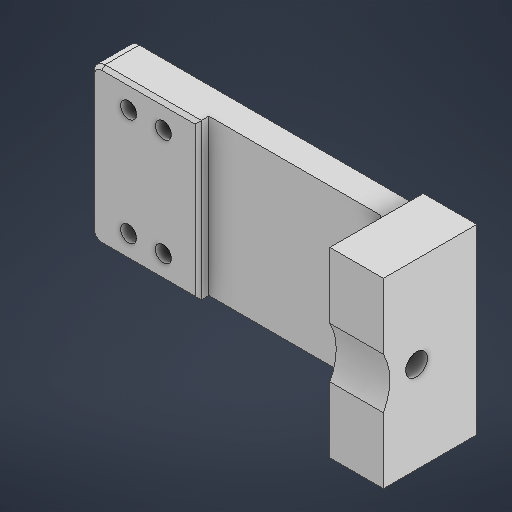
# Autodesk Inventor part: tool4_2
Saved by Autodesk Inventor 2027.1 (Build 311270010, 270A)
## iProperties
Created: 2026-08-16
Part Number: tool4_2
Material: Generic
Document SubType Name: Sheet Metal
Designer: MSI
Density: 1 g/cm^3
Sheet Metal Rule: Default_mm
Appearance: Default
Author: MSI
Autodesk Inventor part; units mm, degrees
ref_plane "YZ Plane" through (0, 0, 0) normal (1, 0, 0) x (0, 1, 0)
ref_plane "XZ Plane" through (0, 0, 0) normal (0, 1, 0) x (-1, 0, 0)
ref_plane "XY Plane" through (0, 0, 0) normal (0, 0, 1) x (1, 0, 0)
sketch "Sketch1" plane through (0, 0, 0) normal (0, 0, 1) x (1, 0, 0)
  line L0 (2, 0) -> (65, 0)
  line L1 (65, 0) -> (65, 29)
  line L2 (65, 29) -> (2, 29)
  line L3 (0, 27) -> (0, 2)
  arc A0 (2, 29) -> (0, 27) centre (2, 27) ccw
  arc A1 (0, 2) -> (2, 0) centre (2, 2) ccw
  line L4 (20, 29) -> (20, 0)
  line L5 (55, 29) -> (55, 0)
  circle A2 centre (7, 24.5) radius 1.5
  circle A3 centre (7, 4.5) radius 1.5
  circle A4 centre (13.5, 24.5) radius 1.5
  circle A5 centre (13.5, 4.5) radius 1.5
  line L6 (65, 0) -> (65, -2.5)
  line L7 (65, -2.5) -> (55, -2.5)
  line L8 (55, -2.5) -> (55, 0)
  line L9 (55, 29) -> (55, 31.5)
  line L10 (55, 31.5) -> (65, 31.5)
  line L11 (65, 31.5) -> (65, 29)
  point P0 (0, 0)
  point P1 (0, 29)
  dimension "d0" = 65
  dimension "d1" = 29
  dimension "d2" = 2
  dimension "d3" = 20
  dimension "d4" = 10
  dimension "d5" = 3
  dimension "d6" = 3
  dimension "d7" = 4.5
  dimension "d8" = 4.5
  dimension "d9" = 20
  dimension "d10" = 3
  dimension "d11" = 3
  dimension "d12" = 20
  dimension "d13" = 6.5
  dimension "d14" = 7
  dimension "d24" = 2.5
  dimension "d25" = 2.5
  constraints: 24 end point, 10 point on line, 7 perpendicular, 6 centre point, 4 point on circle, 4 tangent, 2 parallel, 1 equal radius, 1 horizontal, 1 vertical
  measures "d0" distance of point (0, 29) L1.end
  measures "d1" distance of L0.end L1.end
  measures "d2" radius of A0
  measures "d3" distance from line of L4 L3.end
  measures "d4" distance between parallel lines of L1 L5
  measures "d5" diameter of A2
  measures "d6" diameter of A3
  measures "d7" distance from line of L2 A2.centre
  measures "d8" distance from line of L0 A3.centre
  measures "d9" distance of A3.centre A2.centre
  measures "d10" diameter of A4
  measures "d11" diameter of A5
  measures "d12" distance of A5.centre A4.centre
  measures "d13" distance of A4.centre A2.centre
  measures "d14" distance from line of L3 A2.centre
  measures "d24" distance of L0.end L6.end
  measures "d25" distance of L5.start L9.end
extrude "Extrusion1" add sketch "Sketch1" along normal blind 5 contours L4 L2 L5 L0
extrude "Extrusion2" add sketch "Sketch1" along normal blind 7 contours A1 L3 A0 L2 L4 L0
extrude "Extrusion3" add sketch "Sketch1" along normal blind 26.25 contours L5 L2 L1 L0
sketch "Sketch2" plane through (55, 0, 5) normal (-1, 0, 0) x (0, 0, 1)
  line L0 (21.25, 29) -> (21.25, 0) projected
  circle A0 centre (21.25, 14.5) radius 10
  point P0 (-5, 0)
  point P1 (21.25, 4.5)
  point P2 (21.25, 24.5)
  dimension "d21" = 20
  constraints: 1 centre point, 1 midpoint
  measures "d21" diameter of A0
extrude "Extrusion4" cut sketch "Sketch2" against normal blind 20 contours L0 A0 picked at (15.0351, 13.318)
extrude "Extrusion5" add sketch "Sketch1" along normal blind 26.25 contours L0 L6 L7 L8 | L9 L10 L11 L2
chamfer "Chamfer1" distance 2.5 angle 45 1 edges at (55, 0, 2.5)
chamfer "Chamfer2" distance 2.5 angle 45 1 edges at (55, 29, 2.5)
chamfer "Chamfer4" distance 0.6 angle 45 6 edges at (20, 14.5, 7) (11, 0, 7) (0.5858, 0.5858, 7) (0, 14.5, 7) (0.5858, 28.4142, 7) (11, 29, 7)
sketch "Sketch5" plane through (55, 14.5, 26.25) normal (-1, 0, 0) x (0, 0, 1)
  circle A0 centre (-15, 0) radius 2.05
  line L0 (0, -10) -> (0, -17) projected
  point P0 (-26.25, -14.5)
  dimension "d48" = 4.1
  dimension "d49" = 15
  constraints: 1 centre point
  measures "d48" diameter of A0
  measures "d49" distance from line of L0 A0.centre
extrude "Extrusion7" cut sketch "Sketch5" against normal blind 26.25
extrude "Extrusion8" cut sketch "Sketch5" along normal blind 26.25
sketch "Sketch6" plane through (55, 14.5, 26.25) normal (-1, 0, 0) x (0, 0, 1)
  line L0 (0, 17) -> (0, 10) projected
  line L1 (-21.25, -17) -> (0, -17) projected
  line L2 (0, 17) -> (-8.8131, 17)
  line L3 (-8.8131, 17) -> (-8.8131, -17)
  line L4 (-8.8131, -17) -> (0, -17)
  line L5 (0, -17) -> (0, 17)
  point P0 (-26.25, -14.5)
  point P1 (-15.25, -17)
  constraints: 8 end point, 2 parallel, 1 horizontal, 1 perpendicular, 1 point on line
extrude "Extrusion9" cut sketch "Sketch6" against normal blind 26.25
chamfer "Chamfer5" distance 3 angle 45 1 edges at (55, 14.5, 5)
equation "\"BendRadius\" = Thickness"
equation "\"BendReliefWidth\" = Thickness"
equation "\"BendReliefDepth\" = 0.5 * Thickness"
equation "\"CornerReliefSize\" = 4 * Thickness"
equation "\"MinimumRemnant\" = 2 * Thickness"
equation "\"TransitionRadius\" = BendRadius"
equation "\"JacobiRadiusSize\" = BendRadius"
equation "\"GapSize\" = Thickness"
equation "\"Thickness\" = 0.5"
body "Solid1"
